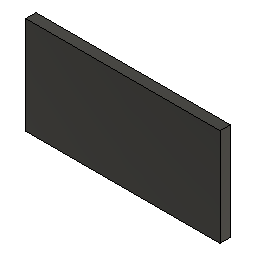
2278 RGB matrix 4mm (Autodesk Fusion 360 design; units mm, degrees)
Autodesk Fusion 360 part; units mm, degrees
sketch "Sketch1" plane through (0, 0, 0) normal (0, 1, 0) x (1, 0, 0)
  line L0 (-127.5, -64) -> (127.5, -64)
  line L1 (127.5, -64) -> (127.5, 64)
  line L2 (127.5, 64) -> (-127.5, 64)
  line L3 (-127.5, 64) -> (-127.5, -64)
  line L4 (127.5, 0) -> (0, 0) construction
  line L5 (0, 0) -> (0, -64) construction
  circle A0 centre (0, -56) radius 2
  circle A1 centre (119.5, -56) radius 2
  circle A2 centre (119.5, 56) radius 2
  circle A3 centre (0, 56) radius 2
  line L6 (119.5, -56) -> (119.5, 56) construction
  circle A4 centre (-119.5, -56) radius 2
  circle A5 centre (-119.5, 56) radius 2
  line L7 (115.5, -52) -> (6.5, -52)
  line L8 (6.5, -52) -> (6.5, 52)
  line L9 (6.5, 52) -> (115.5, 52)
  line L10 (115.5, 52) -> (115.5, -52)
  line L11 (-6.5, 52) -> (-115.5, 52)
  line L12 (-115.5, 52) -> (-115.5, -52)
  line L13 (-115.5, -52) -> (-6.5, -52)
  line L14 (-6.5, -52) -> (-6.5, 52)
  line L15 (115.5, -20) -> (121.5, -20)
  line L16 (121.5, -20) -> (121.5, 20)
  line L17 (121.5, 20) -> (115.5, 20)
  line L18 (121.5, 0) -> (127.5, 0) construction
  line L19 (-115.5, -20) -> (-121.5, -20)
  line L20 (-121.5, -20) -> (-121.5, 20)
  line L21 (-121.5, 20) -> (-115.5, 20)
  dimension "d4" = 255
  dimension "d5" = 128
  dimension "d8" = 4
  dimension "d9" = 8
  dimension "d10" = 4
  dimension "d11" = 8
  dimension "d12" = 8
  dimension "d13" = 12
  dimension "d14" = 12
  dimension "d15" = 6.5
  dimension "d16" = 12
  dimension "d21" = 40
  dimension "d23" = 6
  constraint horizontal L0
  constraint vertical L1
  constraint horizontal L2
  constraint vertical L3
  constraint midpoint L1 L4.start
  constraint coincident L4.end L5.start
  constraint midpoint L0 L5.end
  constraint vertical L5
  constraint horizontal L4
  constraint coincident L5 A0.centre
  constraint symmetric L4 A1 A2
  constraint symmetric L4 A0 A3
  constraint coincident A1.centre L6.start
  constraint coincident A2.centre L6.end
  constraint symmetric L5 A1 A4
  constraint symmetric L5 A2 A5
  constraint horizontal L7
  constraint vertical L8
  constraint horizontal L9
  constraint vertical L10
  constraint symmetric L5 L7.start L12.end
  constraint symmetric L5 L7.end L13.end
  constraint symmetric L5 L8.end L11.start
  constraint symmetric L5 L9.end L11.end
  constraint coincident L10 L15.start
  constraint parallel L10 L16
  constraint coincident L10 L17.end
  constraint perpendicular L16 L17
  constraint perpendicular L15 L16
  constraint midpoint L16 L18.start
  constraint horizontal L18
  constraint symmetric L5 L15.start L19.start
  constraint symmetric L5 L15.end L19.end
  constraint symmetric L5 L16.end L20.end
  constraint symmetric L5 L17.end L21.end
  measures "d4" distance of L0.start L0.end
  measures "d5" distance of L0.end L1.end
  measures "d8" diameter of A0
  measures "d9" distance of L0 A0.centre
  measures "d10" diameter of A1
  measures "d11" distance of L0 A1.centre
  measures "d12" distance of L1 A1.centre
  measures "d13" distance of L0 L7
  measures "d14" distance of L1 L10
  measures "d15" distance of L5 L8
  measures "d16" distance of L2 L9
  measures "d21" distance of L15.end L16.end
  measures "d23" distance of L1 L16
extrude "Extrude1" add sketch "Sketch1" against normal blind 13.5 contours L0 L1 L2 L3 | A0 | A1 | A2 | A3 | A4 | A5 | L7 L8 L9 L10 | L10 L15 L16 L17 | L11 L12 L13 L14 | L12 L19 L20 L21
extrude "Extrude2" cut sketch "Sketch1" against normal blind 10 contours L7 L8 L9 L10 | L10 L15 L16 L17 | L11 L12 L13 L14 | L12 L19 L20 L21
extrude "Extrude3" cut sketch "Sketch1" against normal blind 10 contours A0 | A1 | A2 | A3 | A4 | A5
fillet "Fillet1" radius 3 16 edges at (115.5, -5, -52) (6.5, -5, -52) (6.5, -5, 52) (115.5, -5, 52) (115.5, -5, 20) (121.5, -5, 20) (121.5, -5, -20) (115.5, -5, -20) (-6.5, -5, 52) (-6.5, -5, -52) (-115.5, -5, -52) (-115.5, -5, -20) (-121.5, -5, -20) (-121.5, -5, 20) (-115.5, -5, 20) (-115.5, -5, 52)
equation "matrixWidth = 128 mm"
equation "matrixLength = 255 mm"
equation "matrixThickness = 13.5 mm"
equation "d4 = matrixLength"
equation "d5 = matrixWidth"
equation "d6 = -matrixThickness"
equation "d8 = mHole"
equation "d9 = HoleDist"
equation "d10 = mHole"
equation "d11 = HoleDist"
equation "d12 = HoleDist"
equation "mHole = 4 mm"
equation "HoleDist = 8 mm"
